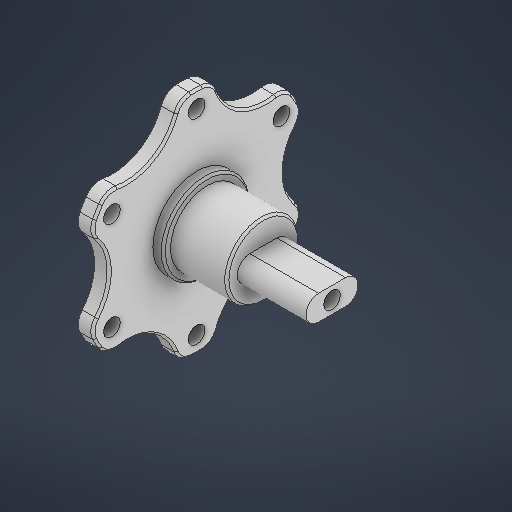
# Autodesk Inventor part: Spindle_CV_Flange_V2
Saved by Autodesk Inventor 2026.1 (Build 301233000, 233)
## iProperties
Created: 2026-09-11
Part Number: Spindle_CV_Flange_V2
Material: Generic
Document SubType Name: Modeling
Designer: share
Density: 1 g/cm^3
Appearance: Default
Author: share
Autodesk Inventor part; units mm, degrees
ref_plane "YZ Plane" through (0, 0, 0) normal (1, 0, 0) x (0, 1, 0)
ref_plane "XZ Plane" through (0, 0, 0) normal (0, 1, 0) x (-1, 0, 0)
ref_plane "XY Plane" through (0, 0, 0) normal (0, 0, 1) x (1, 0, 0)
sketch "Sketch2" plane through (0, 0, 0) normal (1, 0, 0) x (0, 1, 0)
  circle A0 centre (0, 0) radius 55
  circle A1 centre (0, 0) radius 47 construction
  line L0 (0, 0) -> (47, 0) construction
  dimension "d4" = 94
  dimension "d3" = 110
  constraints: 3 coincident, 2 end point, 1 centre point, 1 horizontal, 1 horizontal alignment, 2 other
  measures "d3" diameter of A0
extrude "Flange Main Body" add sketch "Sketch2" along normal blind 8
hole "CV Interface Holes" at (0, 47, 0) direction (1, 0, 0) diameter 8 end through all
pattern_circular "CV Bolt Pattern" count 6 over 360 about axis through (-10, 0, 0) along (1, 0, 0) of "CV Interface Holes"
sketch "Sketch3" plane through (8, 0, 0) normal (1, 0, 0) x (0, 0, -1)
  circle A0 centre (0, 0) radius 21
  dimension "d18" = 42
  constraints: 1 centre point, 1 coincident
  measures "d18" diameter of A0
extrude "Bearing Ring Seat" add sketch "Sketch3" along normal blind 5
sketch "Sketch4" plane through (13, 0, 0) normal (1, 0, 0) x (0, 0, -1)
  circle A0 centre (0, 0) radius 17.5
  dimension "d21" = 35
  constraints: 1 centre point, 1 coincident
  measures "d21" diameter of A0
extrude "Axle" add sketch "Sketch4" along normal blind 60
sketch "Sketch5" plane through (0, 0, 0) normal (-1, 0, 0) x (0, 0, 1)
  point P0 (0, 0)
  point P1 (0, 0)
  constraints: 1 coincident
hole "Axle Bolt Hole" at (0, 0, 0) direction (1, 0, 0) diameter 8 end through all
sketch "Sketch6" plane through (0, 0, 0) normal (-1, 0, 0) x (0, 0, 1)
  circle A0 centre (0, 0) radius 11
  circle A1 centre (0, 0) radius 4 projected
  dimension "d32" = 22
  constraints: 1 centre point, 1 coincident
  measures "d32" diameter of A0
extrude "Axle Bolt Heat Seat" cut sketch "Sketch6" against normal blind 4
sketch "Sketch7" plane through (0, 0, 0) normal (-1, 0, 0) x (0, 0, 1)
  circle A0 centre (0, 0) radius 11 projected
  circle A1 centre (-40.7032, 23.5) radius 4 projected
  circle A2 centre (-40.7032, -23.5) radius 4 projected
  circle A3 centre (0, -47) radius 4 projected
  circle A4 centre (40.7032, -23.5) radius 4 projected
  circle A5 centre (40.7032, 23.5) radius 4 projected
  circle A6 centre (0, 47) radius 4 projected
  circle A7 centre (0, 0) radius 55 projected
  line L0 (-77, 0) -> (77, 0) construction
  line L1 (0, 77) -> (0, -77) construction
  arc A8 (-51.4104, -19.5439) -> (-51.4104, 19.5439) centre (-67, 0) ccw
  dimension "d35" = 25
  dimension "d36" = 67
  constraints: 4 point on circle, 1 centre point, 1 point on line
  measures "d35" radius of A8
  measures "d36" distance from line of L1 A8.centre
extrude "CV Flange Weight Reduction" cut sketch "Sketch7" against normal up to surface (8 mm away) contours A8 A7 picked at (-50.5739, -5.1659)
pattern_circular "CV Flange WR Pattern" count 6 over 360 about axis through (-10, 0, 0) along (1, 0, 0) of "CV Flange Weight Reduction"
fillet "CV Flange WR Fillet" radius 8 12 edges at (4, 19.5439, -51.4104) (4, 34.7508, -42.6308) (4, -19.5439, -51.4104) (4, -34.7508, -42.6308) (4, -54.2947, -8.7797) (4, -54.2947, 8.7797) (4, -34.7508, 42.6308) (4, -19.5439, 51.4104) (4, 19.5439, 51.4104) (4, 34.7508, 42.6308) (4, 54.2947, 8.7797) (4, 54.2947, -8.7797)
sketch "Sketch8" plane through (73, 0, 0) normal (1, 0, 0) x (0, 0, -1)
  circle A0 centre (0, 0) radius 4 projected
  circle A1 centre (0, 0) radius 17.5 projected
  line L0 (-77, 0) -> (77, 0) construction
  line L1 (0, -77) -> (0, 77) construction
  line L2 (-12.5, 6) -> (12.5, 6)
  line L3 (12.5, 6) -> (12.5, -6)
  line L4 (12.5, -6) -> (-12.5, -6)
  line L5 (-12.5, -6) -> (-12.5, 6)
  dimension "d48" = 25
  dimension "d49" = 12
  constraints: 8 end point, 2 parallel, 1 horizontal, 1 perpendicular, 2 other
  measures "d48" distance between parallel lines of L3 L5
  measures "d49" distance between parallel lines of L4 L2
extrude "Wheel Hub Rectangle" cut sketch "Sketch8" against normal blind 33 contours A1
fillet "WHR Fillet" radius 6 4 edges at (56.5, 6, 12.5) (56.5, -6, 12.5) (56.5, -6, -12.5) (56.5, 6, -12.5)
chamfer "Chamfer1" distance 1 angle 45 50 edges at (13, 0, 21) (40, 0, 17.5) (8, 0, 42) (8, -20.4472, 49.8042) (8, -27.5, 47.6314) (8, -32.9081, 42.61) (8, -36.3731, 21) (8, -53.3553, 7.1943) (8, -55, 0) (8, -53.3554, -7.1943) (8, -36.3731, -21) (8, -32.9081, -42.6099) (8, -27.5, -47.6314) (8, -20.4473, -49.8042) (8, 0, -42) (8, 20.4473, -49.8042) (8, 27.5, -47.6314) (8, 32.9081, -42.6099) (8, 36.3731, -21) (8, 53.3553, -7.1943) (8, 55, 0) (8, 53.3554, 7.1943) (8, 36.3731, 21) (8, 32.9081, 42.6099) (8, 27.5, 47.6314) (8, 20.4473, 49.8042) (0, 0, 42) (0, 20.4473, 49.8042) (0, 27.5, 47.6314) (0, 32.9081, 42.6099) (0, 36.3731, 21) (0, 53.3554, 7.1943) (0, 55, 0) (0, 53.3553, -7.1943) (0, 36.3731, -21) (0, 32.9081, -42.61) (0, 27.5, -47.6314) (0, 20.4473, -49.8042) (0, 0, -42) (0, -20.4473, -49.8042) (0, -27.5, -47.6314) (0, -32.9081, -42.6099) (0, -36.3731, -21) (0, -53.3554, -7.1943) (0, -55, 0) (0, -53.3553, 7.1943) (0, -36.3731, 21) (0, -32.9081, 42.61) (0, -27.5, 47.6314) (0, -20.4472, 49.8042)
body "Solid1"
